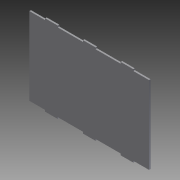
# Autodesk Inventor part: it shelf
Saved by Autodesk Inventor 2011 (Build 150239000, 239)
## iProperties
Created: 2011-09-10
Part Number: it shelf
Document SubType Name: Modeling
Designer: Matthew
Density: 1 g/cm^3
Author: Matthew
Autodesk Inventor part; units mm, degrees
ref_plane "YZ Plane" through (0, 0, 0) normal (1, 0, 0) x (0, 1, 0)
ref_plane "XZ Plane" through (0, 0, 0) normal (0, 1, 0) x (-1, 0, 0)
ref_plane "XY Plane" through (0, 0, 0) normal (0, 0, 1) x (1, 0, 0)
sketch "Sketch1" plane through (0, 0, 0) normal (0, 0, 1) x (1, 0, 0)
  line L0 (-26.4658, 20.5619) -> (456.1342, 20.5619)
  line L1 (456.1342, 20.5619) -> (456.1342, -293.1281)
  line L2 (456.1342, -293.1281) -> (-26.4658, -293.1281)
  line L3 (-26.4658, -293.1281) -> (-26.4658, 20.5619)
  line L4 (-26.4658, 20.5619) -> (37.0342, 20.5619)
  line L5 (37.0342, 20.5619) -> (87.8342, 20.5619)
  line L6 (87.8342, 20.5619) -> (189.4342, 20.5619)
  line L7 (189.4342, 20.5619) -> (240.2342, 20.5619)
  line L8 (240.2342, 20.5619) -> (341.8342, 20.5619)
  line L9 (341.8342, 20.5619) -> (392.6342, 20.5619)
  line L10 (392.6342, 20.5619) -> (456.1342, 20.5619)
  line L11 (37.0342, 20.5619) -> (87.8342, 20.5619)
  line L12 (87.8342, 20.5619) -> (87.8342, 26.9119)
  line L13 (87.8342, 26.9119) -> (37.0342, 26.9119)
  line L14 (37.0342, 26.9119) -> (37.0342, 20.5619)
  line L15 (189.4342, 20.5619) -> (240.2342, 20.5619)
  line L16 (240.2342, 20.5619) -> (240.2342, 26.9119)
  line L17 (240.2342, 26.9119) -> (189.4342, 26.9119)
  line L18 (189.4342, 26.9119) -> (189.4342, 20.5619)
  line L19 (341.8342, 20.5619) -> (392.6342, 20.5619)
  line L20 (392.6342, 20.5619) -> (392.6342, 26.9119)
  line L21 (392.6342, 26.9119) -> (341.8342, 26.9119)
  line L22 (341.8342, 26.9119) -> (341.8342, 20.5619)
  line L23 (37.0342, -293.1281) -> (87.8342, -293.1281)
  line L24 (87.8342, -293.1281) -> (87.8342, -299.4781)
  line L25 (87.8342, -299.4781) -> (37.0342, -299.4781)
  line L26 (37.0342, -299.4781) -> (37.0342, -293.1281)
  line L27 (189.4342, -293.1281) -> (240.2342, -293.1281)
  line L28 (240.2342, -293.1281) -> (240.2342, -299.4781)
  line L29 (240.2342, -299.4781) -> (189.4342, -299.4781)
  line L30 (189.4342, -299.4781) -> (189.4342, -293.1281)
  line L31 (341.8342, -293.1281) -> (392.6342, -293.1281)
  line L32 (392.6342, -293.1281) -> (392.6342, -299.4781)
  line L33 (392.6342, -299.4781) -> (341.8342, -299.4781)
  line L34 (341.8342, -299.4781) -> (341.8342, -293.1281)
  point P0 (0, 0)
  dimension "d0" = 482.6
  dimension "d1" = 313.69
  dimension "d2" = 63.5
  dimension "d3" = 50.8
  dimension "d4" = 101.6
  dimension "d5" = 50.8
  dimension "d6" = 101.6
  dimension "d7" = 50.8
  dimension "d8" = 63.5
  dimension "d9" = 6.35
  dimension "d10" = 6.35
  constraints: 70 end point, 14 parallel, 9 point on line, 7 horizontal, 7 perpendicular, 1 collinear
  measures "d0" distance of L1.end L2.end
  measures "d1" distance of L0.end L1.end
  measures "d2" distance of L0.start L4.end
  measures "d3" distance of L4.end L5.end
  measures "d4" distance of L5.end L6.end
  measures "d5" distance of L6.end L7.end
  measures "d6" distance of L7.end L8.end
  measures "d7" distance of L8.end L9.end
  measures "d8" distance of L9.end L0.end
  measures "d9" distance of L12.end L11.end
  measures "d10" distance of L23.end L24.end
extrude "Extrusion1" add sketch "Sketch1" along normal blind 6.35
body "Solid1"
